Autodesk Fusion 360 part; units mm, degrees
(part 3 of 8)
  spline S114 degree 5 poles (48.8425, -65.8666) (48.8377, -65.8463) (48.8283, -65.8055) (48.814, -65.7444) (48.7948, -65.663) (48.7704, -65.5615) (48.7458, -65.4601) (48.7208, -65.3589) (48.6955, -65.2578) (48.6699, -65.1568) (48.644, -65.0561) (48.6178, -64.9555) (48.5912, -64.855) (48.5643, -64.7547) (48.5371, -64.6546) (48.5096, -64.5547) (48.4817, -64.4549) (48.4535, -64.3553) (48.4249, -64.2559) (48.396, -64.1566) (48.3668, -64.0575) (48.3373, -63.9587) (48.3074, -63.86) (48.2771, -63.7614) (48.2465, -63.6631) (48.2156, -63.565) (48.1842, -63.467) (48.1526, -63.3693) (48.1206, -63.2717) (48.0882, -63.1744) (48.0554, -63.0772) (48.0223, -62.9803) (47.9888, -62.8835) (47.9549, -62.787) (47.9207, -62.6907) (47.8861, -62.5946) (47.851, -62.4988) (47.8156, -62.4032) (47.7852, -62.322) (47.7617, -62.2601) (47.7453, -62.2173) (47.7362, -62.1935) (47.7343, -62.1887) knots -1 -1 -1 -1 -1 -1 -0.985714 -0.971429 -0.957143 -0.942857 -0.928571 -0.914286 -0.9 -0.885714 -0.871429 -0.857143 -0.842857 -0.828571 -0.814286 -0.8 -0.785714 -0.771429 -0.757143 -0.742857 -0.728571 -0.714286 -0.7 -0.685714 -0.671429 -0.657143 -0.642857 -0.628571 -0.614286 -0.6 -0.585714 -0.571429 -0.557143 -0.542857 -0.528571 -0.514286 -0.5 -0.485714 -0.471429 -0.467834 -0.467834 -0.467834 -0.467834 -0.467834 -0.467834
  spline S115 degree 3 poles (48.0492, -61.0441) (47.9469, -61.1247) (47.8613, -61.2244) (47.7331, -61.4511) (47.6918, -61.5759) (47.6653, -61.7866) (47.6651, -61.869) (47.6849, -62.0321) (47.7049, -62.1121) (47.7343, -62.1887) knots 0 0 0 0 0.039064 0.039064 0.078129 0.078129 0.102767 0.102767 0.127404 0.127404 0.127404 0.127404
  arc A58 (48.0492, -61.0441) -> (48.1406, -60.9721) centre (0, 0) ccw
  spline S116 degree 3 poles (49.3271, -60.9331) (49.2198, -60.8593) (49.0992, -60.8071) (48.8446, -60.752) (48.7132, -60.7496) (48.5041, -60.7868) (48.4254, -60.8111) (48.2756, -60.8784) (48.2051, -60.9212) (48.1406, -60.9721) knots 0 0 0 0 0.039064 0.039064 0.078129 0.078129 0.102767 0.102767 0.127404 0.127404 0.127404 0.127404
  spline S117 degree 5 poles (49.3271, -60.9331) (49.3313, -60.936) (49.3523, -60.9504) (49.3901, -60.9764) (49.4448, -61.0137) (49.5166, -61.0622) (49.6013, -61.119) (49.6864, -61.1754) (49.7717, -61.2315) (49.8574, -61.2873) (49.9433, -61.3427) (50.0295, -61.3979) (50.1161, -61.4527) (50.2029, -61.5073) (50.29, -61.5615) (50.3774, -61.6154) (50.465, -61.669) (50.553, -61.7223) (50.6412, -61.7753) (50.7296, -61.828) (50.8184, -61.8804) (50.9074, -61.9325) (50.9966, -61.9844) (51.0861, -62.0359) (51.1759, -62.0872) (51.2659, -62.1381) (51.3562, -62.1888) (51.4467, -62.2392) (51.5374, -62.2893) (51.6284, -62.3392) (51.7197, -62.3887) (51.8111, -62.438) (51.9028, -62.487) (51.9948, -62.5357) (52.0869, -62.5842) (52.1793, -62.6324) (52.2719, -62.6803) (52.3648, -62.7279) (52.4579, -62.7753) (52.5325, -62.813) (52.5886, -62.8411) (52.626, -62.8599) (52.6447, -62.8692) knots 0.467834 0.467834 0.467834 0.467834 0.467834 0.467834 0.471429 0.485714 0.5 0.514286 0.528571 0.542857 0.557143 0.571429 0.585714 0.6 0.614286 0.628571 0.642857 0.657143 0.671429 0.685714 0.7 0.714286 0.728571 0.742857 0.757143 0.771429 0.785714 0.8 0.814286 0.828571 0.842857 0.857143 0.871429 0.885714 0.9 0.914286 0.928571 0.942857 0.957143 0.971429 0.985714 1 1 1 1 1 1
  arc A59 (52.6447, -62.8692) -> (53.8597, -61.8315) centre (0, 0) ccw
  spline S118 degree 5 poles (53.8597, -61.8315) (53.8534, -61.8115) (53.8408, -61.7716) (53.8218, -61.7118) (53.7962, -61.6322) (53.764, -61.5329) (53.7315, -61.4338) (53.6986, -61.3348) (53.6655, -61.236) (53.632, -61.1374) (53.5983, -61.039) (53.5642, -60.9407) (53.5299, -60.8427) (53.4952, -60.7448) (53.4602, -60.6471) (53.4249, -60.5497) (53.3893, -60.4524) (53.3534, -60.3553) (53.3171, -60.2584) (53.2805, -60.1617) (53.2436, -60.0653) (53.2064, -59.969) (53.1688, -59.8729) (53.1309, -59.7771) (53.0927, -59.6815) (53.0542, -59.5861) (53.0153, -59.4909) (52.976, -59.3959) (52.9365, -59.3012) (52.8965, -59.2067) (52.8563, -59.1124) (52.8156, -59.0183) (52.7747, -58.9245) (52.7333, -58.831) (52.6916, -58.7377) (52.6496, -58.6446) (52.6071, -58.5518) (52.5643, -58.4592) (52.5276, -58.3807) (52.4993, -58.3209) (52.4796, -58.2795) (52.4687, -58.2565) (52.4665, -58.2518) knots -1 -1 -1 -1 -1 -1 -0.985714 -0.971429 -0.957143 -0.942857 -0.928571 -0.914286 -0.9 -0.885714 -0.871429 -0.857143 -0.842857 -0.828571 -0.814286 -0.8 -0.785714 -0.771429 -0.757143 -0.742857 -0.728571 -0.714286 -0.7 -0.685714 -0.671429 -0.657143 -0.642857 -0.628571 -0.614286 -0.6 -0.585714 -0.571429 -0.557143 -0.542857 -0.528571 -0.514286 -0.5 -0.485714 -0.471429 -0.467834 -0.467834 -0.467834 -0.467834 -0.467834 -0.467834
  spline S119 degree 3 poles (52.6906, -57.0861) (52.5949, -57.1744) (52.5174, -57.2805) (52.4074, -57.5166) (52.376, -57.6443) (52.3661, -57.8564) (52.3724, -57.9386) (52.4049, -58.0996) (52.4311, -58.1777) (52.4665, -58.2518) knots 0 0 0 0 0.039064 0.039064 0.078129 0.078129 0.102767 0.102767 0.127404 0.127404 0.127404 0.127404
  arc A60 (52.6906, -57.0861) -> (52.776, -57.0071) centre (0, 0) ccw
  spline S120 degree 3 poles (53.9558, -56.8751) (53.8431, -56.8099) (53.7187, -56.7674) (53.4606, -56.7325) (53.3294, -56.7403) (53.1239, -56.7938) (53.0473, -56.8243) (52.9032, -56.9031) (52.8363, -56.9513) (52.776, -57.0071) knots 0 0 0 0 0.039064 0.039064 0.078129 0.078129 0.102767 0.102767 0.127404 0.127404 0.127404 0.127404
  spline S121 degree 5 poles (53.9558, -56.8751) (53.9602, -56.8777) (53.9823, -56.8904) (54.022, -56.9133) (54.0795, -56.9462) (54.1549, -56.9889) (54.2438, -57.0389) (54.333, -57.0885) (54.4224, -57.1377) (54.5122, -57.1866) (54.6022, -57.2351) (54.6925, -57.2834) (54.7831, -57.3312) (54.8739, -57.3788) (54.965, -57.426) (55.0564, -57.4729) (55.148, -57.5194) (55.2398, -57.5657) (55.3319, -57.6116) (55.4242, -57.6572) (55.5168, -57.7025) (55.6096, -57.7475) (55.7027, -57.7922) (55.7959, -57.8365) (55.8894, -57.8806) (55.9832, -57.9243) (56.0771, -57.9678) (56.1713, -58.0109) (56.2657, -58.0537) (56.3604, -58.0963) (56.4552, -58.1385) (56.5503, -58.1805) (56.6455, -58.2221) (56.741, -58.2635) (56.8367, -58.3046) (56.9326, -58.3454) (57.0287, -58.3859) (57.1249, -58.4261) (57.2214, -58.466) (57.2988, -58.4977) (57.3569, -58.5214) (57.3957, -58.5371) (57.4151, -58.5449) knots 0.467834 0.467834 0.467834 0.467834 0.467834 0.467834 0.471429 0.485714 0.5 0.514286 0.528571 0.542857 0.557143 0.571429 0.585714 0.6 0.614286 0.628571 0.642857 0.657143 0.671429 0.685714 0.7 0.714286 0.728571 0.742857 0.757143 0.771429 0.785714 0.8 0.814286 0.828571 0.842857 0.857143 0.871429 0.885714 0.9 0.914286 0.928571 0.942857 0.957143 0.971429 0.985714 1 1 1 1 1 1
  arc A61 (57.4151, -58.5449) -> (58.5449, -57.4151) centre (0, 0) ccw
  spline S122 degree 5 poles (58.5449, -57.4151) (58.5371, -57.3957) (58.5214, -57.3569) (58.4977, -57.2988) (58.466, -57.2214) (58.4261, -57.1249) (58.3859, -57.0287) (58.3454, -56.9326) (58.3046, -56.8367) (58.2635, -56.741) (58.2221, -56.6455) (58.1805, -56.5503) (58.1385, -56.4552) (58.0963, -56.3604) (58.0537, -56.2657) (58.0109, -56.1713) (57.9678, -56.0771) (57.9243, -55.9832) (57.8806, -55.8894) (57.8365, -55.7959) (57.7922, -55.7027) (57.7475, -55.6096) (57.7025, -55.5168) (57.6572, -55.4242) (57.6116, -55.3319) (57.5657, -55.2398) (57.5194, -55.148) (57.4729, -55.0564) (57.426, -54.965) (57.3788, -54.8739) (57.3312, -54.7831) (57.2834, -54.6925) (57.2351, -54.6022) (57.1866, -54.5122) (57.1377, -54.4224) (57.0885, -54.333) (57.0389, -54.2438) (56.9889, -54.1549) (56.9462, -54.0795) (56.9133, -54.022) (56.8904, -53.9823) (56.8777, -53.9602) (56.8751, -53.9558) knots -1 -1 -1 -1 -1 -1 -0.985714 -0.971429 -0.957143 -0.942857 -0.928571 -0.914286 -0.9 -0.885714 -0.871429 -0.857143 -0.842857 -0.828571 -0.814286 -0.8 -0.785714 -0.771429 -0.757143 -0.742857 -0.728571 -0.714286 -0.7 -0.685714 -0.671429 -0.657143 -0.642857 -0.628571 -0.614286 -0.6 -0.585714 -0.571429 -0.557143 -0.542857 -0.528571 -0.514286 -0.5 -0.485714 -0.471429 -0.467834 -0.467834 -0.467834 -0.467834 -0.467834 -0.467834
  spline S123 degree 3 poles (57.0071, -52.776) (56.9186, -52.8716) (56.8497, -52.9835) (56.7585, -53.2275) (56.7372, -53.3572) (56.744, -53.5694) (56.7567, -53.6509) (56.8018, -53.8088) (56.834, -53.8847) (56.8751, -53.9558) knots 0 0 0 0 0.039064 0.039064 0.078129 0.078129 0.102767 0.102767 0.127404 0.127404 0.127404 0.127404
  arc A62 (57.0071, -52.776) -> (57.0861, -52.6906) centre (0, 0) ccw
  spline S124 degree 3 poles (58.2518, -52.4665) (58.1343, -52.4103) (58.007, -52.3777) (57.747, -52.3631) (57.6168, -52.3812) (57.4161, -52.4507) (57.3421, -52.487) (57.2047, -52.577) (57.1418, -52.6302) (57.0861, -52.6906) knots 0 0 0 0 0.039064 0.039064 0.078129 0.078129 0.102767 0.102767 0.127404 0.127404 0.127404 0.127404
  spline S125 degree 5 poles (58.2518, -52.4665) (58.2565, -52.4687) (58.2795, -52.4796) (58.3209, -52.4993) (58.3807, -52.5276) (58.4592, -52.5643) (58.5518, -52.6071) (58.6446, -52.6496) (58.7377, -52.6916) (58.831, -52.7333) (58.9245, -52.7747) (59.0183, -52.8156) (59.1124, -52.8563) (59.2067, -52.8965) (59.3012, -52.9365) (59.3959, -52.976) (59.4909, -53.0153) (59.5861, -53.0542) (59.6815, -53.0927) (59.7771, -53.1309) (59.8729, -53.1688) (59.969, -53.2064) (60.0653, -53.2436) (60.1617, -53.2805) (60.2584, -53.3171) (60.3553, -53.3534) (60.4524, -53.3893) (60.5497, -53.4249) (60.6471, -53.4602) (60.7448, -53.4952) (60.8427, -53.5299) (60.9407, -53.5642) (61.039, -53.5983) (61.1374, -53.632) (61.236, -53.6655) (61.3348, -53.6986) (61.4338, -53.7315) (61.5329, -53.764) (61.6322, -53.7962) (61.7118, -53.8218) (61.7716, -53.8408) (61.8115, -53.8534) (61.8315, -53.8597) knots 0.467834 0.467834 0.467834 0.467834 0.467834 0.467834 0.471429 0.485714 0.5 0.514286 0.528571 0.542857 0.557143 0.571429 0.585714 0.6 0.614286 0.628571 0.642857 0.657143 0.671429 0.685714 0.7 0.714286 0.728571 0.742857 0.757143 0.771429 0.785714 0.8 0.814286 0.828571 0.842857 0.857143 0.871429 0.885714 0.9 0.914286 0.928571 0.942857 0.957143 0.971429 0.985714 1 1 1 1 1 1
  arc A63 (61.8315, -53.8597) -> (62.8692, -52.6447) centre (0, 0) ccw
  spline S126 degree 5 poles (62.8692, -52.6447) (62.8599, -52.626) (62.8411, -52.5886) (62.813, -52.5325) (62.7753, -52.4579) (62.7279, -52.3648) (62.6803, -52.2719) (62.6324, -52.1793) (62.5842, -52.0869) (62.5357, -51.9948) (62.487, -51.9028) (62.438, -51.8111) (62.3887, -51.7197) (62.3392, -51.6284) (62.2893, -51.5374) (62.2392, -51.4467) (62.1888, -51.3562) (62.1381, -51.2659) (62.0872, -51.1759) (62.0359, -51.0861) (61.9844, -50.9966) (61.9325, -50.9074) (61.8804, -50.8184) (61.828, -50.7296) (61.7753, -50.6412) (61.7223, -50.553) (61.669, -50.465) (61.6154, -50.3774) (61.5615, -50.29) (61.5073, -50.2029) (61.4527, -50.1161) (61.3979, -50.0295) (61.3427, -49.9433) (61.2873, -49.8574) (61.2315, -49.7717) (61.1754, -49.6864) (61.119, -49.6013) (61.0622, -49.5166) (61.0137, -49.4448) (60.9764, -49.3901) (60.9504, -49.3523) (60.936, -49.3313) (60.9331, -49.3271) knots -1 -1 -1 -1 -1 -1 -0.985714 -0.971429 -0.957143 -0.942857 -0.928571 -0.914286 -0.9 -0.885714 -0.871429 -0.857143 -0.842857 -0.828571 -0.814286 -0.8 -0.785714 -0.771429 -0.757143 -0.742857 -0.728571 -0.714286 -0.7 -0.685714 -0.671429 -0.657143 -0.642857 -0.628571 -0.614286 -0.6 -0.585714 -0.571429 -0.557143 -0.542857 -0.528571 -0.514286 -0.5 -0.485714 -0.471429 -0.467834 -0.467834 -0.467834 -0.467834 -0.467834 -0.467834
  spline S127 degree 3 poles (60.9721, -48.1406) (60.8914, -48.2428) (60.8314, -48.3598) (60.7597, -48.6102) (60.7487, -48.7411) (60.7721, -48.9522) (60.7912, -49.0324) (60.8485, -49.1863) (60.8865, -49.2595) (60.9331, -49.3271) knots 0 0 0 0 0.039064 0.039064 0.078129 0.078129 0.102767 0.102767 0.127404 0.127404 0.127404 0.127404
  arc A64 (60.9721, -48.1406) -> (61.0441, -48.0492) centre (0, 0) ccw
  spline S128 degree 3 poles (62.1887, -47.7343) (62.0672, -47.6876) (61.9377, -47.6651) (61.6773, -47.6709) (61.549, -47.6992) (61.3544, -47.7842) (61.2835, -47.8262) (61.1535, -47.9267) (61.0949, -47.9847) (61.0441, -48.0492) knots 0 0 0 0 0.039064 0.039064 0.078129 0.078129 0.102767 0.102767 0.127404 0.127404 0.127404 0.127404
  spline S129 degree 5 poles (62.1887, -47.7343) (62.1935, -47.7362) (62.2173, -47.7453) (62.2601, -47.7617) (62.322, -47.7852) (62.4032, -47.8156) (62.4988, -47.851) (62.5946, -47.8861) (62.6907, -47.9207) (62.787, -47.9549) (62.8835, -47.9888) (62.9803, -48.0223) (63.0772, -48.0554) (63.1744, -48.0882) (63.2717, -48.1206) (63.3693, -48.1526) (63.467, -48.1842) (63.565, -48.2156) (63.6631, -48.2465) (63.7614, -48.2771) (63.86, -48.3074) (63.9587, -48.3373) (64.0575, -48.3668) (64.1566, -48.396) (64.2559, -48.4249) (64.3553, -48.4535) (64.4549, -48.4817) (64.5547, -48.5096) (64.6546, -48.5371) (64.7547, -48.5643) (64.855, -48.5912) (64.9555, -48.6178) (65.0561, -48.644) (65.1568, -48.6699) (65.2578, -48.6955) (65.3589, -48.7208) (65.4601, -48.7458) (65.5615, -48.7704) (65.663, -48.7948) (65.7444, -48.814) (65.8055, -48.8283) (65.8463, -48.8377) (65.8666, -48.8425) knots 0.467834 0.467834 0.467834 0.467834 0.467834 0.467834 0.471429 0.485714 0.5 0.514286 0.528571 0.542857 0.557143 0.571429 0.585714 0.6 0.614286 0.628571 0.642857 0.657143 0.671429 0.685714 0.7 0.714286 0.728571 0.742857 0.757143 0.771429 0.785714 0.8 0.814286 0.828571 0.842857 0.857143 0.871429 0.885714 0.9 0.914286 0.928571 0.942857 0.957143 0.971429 0.985714 1 1 1 1 1 1
  arc A65 (65.8666, -48.8425) -> (66.8058, -47.5498) centre (0, 0) ccw
  spline S130 degree 5 poles (66.8058, -47.5498) (66.7951, -47.5318) (66.7735, -47.496) (66.741, -47.4423) (66.6976, -47.3708) (66.6431, -47.2818) (66.5883, -47.193) (66.5333, -47.1044) (66.478, -47.0161) (66.4224, -46.928) (66.3666, -46.8402) (66.3106, -46.7526) (66.2543, -46.6653) (66.1977, -46.5782) (66.1409, -46.4914) (66.0838, -46.4049) (66.0265, -46.3186) (65.9689, -46.2326) (65.911, -46.1468) (65.8529, -46.0614) (65.7945, -45.9762) (65.7358, -45.8913) (65.6768, -45.8066) (65.6176, -45.7223) (65.5581, -45.6382) (65.4984, -45.5544) (65.4383, -45.471) (65.378, -45.3878) (65.3174, -45.3049) (65.2565, -45.2223) (65.1954, -45.1401) (65.1339, -45.0581) (65.0721, -44.9764) (65.0101, -44.8951) (64.9478, -44.8141) (64.8852, -44.7334) (64.8222, -44.6531) (64.759, -44.5731) (64.705, -44.5053) (64.6635, -44.4537) (64.6347, -44.4181) (64.6186, -44.3983) (64.6154, -44.3943) knots -1 -1 -1 -1 -1 -1 -0.985714 -0.971429 -0.957143 -0.942857 -0.928571 -0.914286 -0.9 -0.885714 -0.871429 -0.857143 -0.842857 -0.828571 -0.814286 -0.8 -0.785714 -0.771429 -0.757143 -0.742857 -0.728571 -0.714286 -0.7 -0.685714 -0.671429 -0.657143 -0.642857 -0.628571 -0.614286 -0.6 -0.585714 -0.571429 -0.557143 -0.542857 -0.528571 -0.514286 -0.5 -0.485714 -0.471429 -0.467834 -0.467834 -0.467834 -0.467834 -0.467834 -0.467834
  spline S131 degree 3 poles (64.5612, -43.2084) (64.4888, -43.3166) (64.4382, -43.4379) (64.3863, -43.6932) (64.3856, -43.8246) (64.4255, -44.0332) (64.4508, -44.1116) (64.52, -44.2606) (64.5637, -44.3305) (64.6154, -44.3943) knots 0 0 0 0 0.039064 0.039064 0.078129 0.078129 0.102767 0.102767 0.127404 0.127404 0.127404 0.127404
  arc A66 (64.5612, -43.2084) -> (64.6259, -43.1116) centre (0, 0) ccw
  spline S132 degree 3 poles (65.7422, -42.7079) (65.6174, -42.6709) (65.4865, -42.6586) (65.2274, -42.6848) (65.1017, -42.7231) (64.9143, -42.8231) (64.8469, -42.8706) (64.7253, -42.9809) (64.6714, -43.0433) (64.6259, -43.1116) knots 0 0 0 0 0.039064 0.039064 0.078129 0.078129 0.102767 0.102767 0.127404 0.127404 0.127404 0.127404
  spline S133 degree 5 poles (65.7422, -42.7079) (65.7471, -42.7094) (65.7716, -42.7166) (65.8155, -42.7296) (65.8791, -42.7481) (65.9624, -42.7721) (66.0605, -42.7999) (66.1588, -42.8273) (66.2573, -42.8543) (66.356, -42.8809) (66.4549, -42.9071) (66.5539, -42.9329) (66.6532, -42.9583) (66.7526, -42.9833) (66.8522, -43.008) (66.9519, -43.0322) (67.0519, -43.0561) (67.152, -43.0797) (67.2522, -43.1028) (67.3527, -43.1256) (67.4532, -43.148) (67.554, -43.1701) (67.6549, -43.1918) (67.756, -43.2132) (67.8572, -43.2342) (67.9585, -43.2548) (68.06, -43.2752) (68.1617, -43.2951) (68.2635, -43.3147) (68.3654, -43.334) (68.4675, -43.353) (68.5697, -43.3716) (68.6721, -43.3898) (68.7746, -43.4078) (68.8772, -43.4254) (68.98, -43.4426) (69.0829, -43.4596) (69.1859, -43.4762) (69.289, -43.4925) (69.3716, -43.5053) (69.4337, -43.5147) (69.475, -43.521) (69.4957, -43.524) knots 0.467834 0.467834 0.467834 0.467834 0.467834 0.467834 0.471429 0.485714 0.5 0.514286 0.528571 0.542857 0.557143 0.571429 0.585714 0.6 0.614286 0.628571 0.642857 0.657143 0.671429 0.685714 0.7 0.714286 0.728571 0.742857 0.757143 0.771429 0.785714 0.8 0.814286 0.828571 0.842857 0.857143 0.871429 0.885714 0.9 0.914286 0.928571 0.942857 0.957143 0.971429 0.985714 1 1 1 1 1 1
  arc A67 (69.4957, -43.524) -> (70.3306, -42.1616) centre (0, 0) ccw
  spline S134 degree 5 poles (70.3306, -42.1616) (70.3185, -42.1446) (70.2941, -42.1106) (70.2576, -42.0596) (70.2087, -41.9918) (70.1473, -41.9073) (70.0857, -41.823) (70.0239, -41.7391) (69.9619, -41.6553) (69.8996, -41.5719) (69.8371, -41.4887) (69.7743, -41.4058) (69.7114, -41.3232) (69.6481, -41.2408) (69.5847, -41.1587) (69.521, -41.0769) (69.457, -40.9954) (69.3929, -40.9142) (69.3285, -40.8333) (69.2638, -40.7526) (69.1989, -40.6723) (69.1337, -40.5922) (69.0683, -40.5125) (69.0027, -40.433) (68.9368, -40.3539) (68.8706, -40.2751) (68.8042, -40.1966) (68.7376, -40.1184) (68.6706, -40.0405) (68.6035, -39.963) (68.536, -39.8857) (68.4683, -39.8088) (68.4004, -39.7323) (68.3321, -39.6561) (68.2636, -39.5802) (68.1949, -39.5047) (68.1258, -39.4296) (68.0565, -39.3548) (67.9974, -39.2915) (67.9519, -39.2433) (67.9204, -39.21) (67.9029, -39.1915) (67.8994, -39.1878) knots -1 -1 -1 -1 -1 -1 -0.985714 -0.971429 -0.957143 -0.942857 -0.928571 -0.914286 -0.9 -0.885714 -0.871429 -0.857143 -0.842857 -0.828571 -0.814286 -0.8 -0.785714 -0.771429 -0.757143 -0.742857 -0.728571 -0.714286 -0.7 -0.685714 -0.671429 -0.657143 -0.642857 -0.628571 -0.614286 -0.6 -0.585714 -0.571429 -0.557143 -0.542857 -0.528571 -0.514286 -0.5 -0.485714 -0.471429 -0.467834 -0.467834 -0.467834 -0.467834 -0.467834 -0.467834
  spline S135 degree 3 poles (67.7523, -38.0098) (67.6886, -38.1234) (67.6476, -38.2483) (67.616, -38.5068) (67.6256, -38.6379) (67.6817, -38.8427) (67.7131, -38.9189) (67.7938, -39.0619) (67.8428, -39.1282) (67.8994, -39.1878) knots 0 0 0 0 0.039064 0.039064 0.078129 0.078129 0.102767 0.102767 0.127404 0.127404 0.127404 0.127404
  arc A68 (67.7523, -38.0098) -> (67.8091, -37.9083) centre (0, 0) ccw
  spline S136 degree 3 poles (68.8904, -37.4182) (68.763, -37.391) (68.6316, -37.389) (68.3754, -37.4355) (68.253, -37.4836) (68.0741, -37.598) (68.0106, -37.6506) (67.898, -37.7701) (67.8492, -37.8366) (67.8091, -37.9083) knots 0 0 0 0 0.039064 0.039064 0.078129 0.078129 0.102767 0.102767 0.127404 0.127404 0.127404 0.127404
  spline S137 degree 5 poles (68.8904, -37.4182) (68.8954, -37.4192) (68.9203, -37.4245) (68.9652, -37.434) (69.03, -37.4475) (69.1149, -37.4649) (69.2149, -37.4849) (69.315, -37.5045) (69.4153, -37.5237) (69.5158, -37.5425) (69.6164, -37.5608) (69.7172, -37.5788) (69.8182, -37.5963) (69.9192, -37.6135) (70.0204, -37.6302) (70.1218, -37.6466) (70.2233, -37.6626) (70.3249, -37.6782) (70.4267, -37.6934) (70.5286, -37.7082) (70.6307, -37.7227) (70.7328, -37.7368) (70.8351, -37.7505) (70.9376, -37.7639) (71.0401, -37.7769) (71.1428, -37.7895) (71.2456, -37.8018) (71.3485, -37.8137) (71.4515, -37.8253) (71.5546, -37.8365) (71.6579, -37.8474) (71.7612, -37.8579) (71.8647, -37.8681) (71.9683, -37.878) (72.072, -37.8875) (72.1758, -37.8966) (72.2797, -37.9054) (72.3837, -37.9139) (72.4878, -37.9221) (72.5712, -37.9283) (72.6338, -37.9329) (72.6755, -37.9358) (72.6964, -37.9373) knots 0.467834 0.467834 0.467834 0.467834 0.467834 0.467834 0.471429 0.485714 0.5 0.514286 0.528571 0.542857 0.557143 0.571429 0.585714 0.6 0.614286 0.628571 0.642857 0.657143 0.671429 0.685714 0.7 0.714286 0.728571 0.742857 0.757143 0.771429 0.785714 0.8 0.814286 0.828571 0.842857 0.857143 0.871429 0.885714 0.9 0.914286 0.928571 0.942857 0.957143 0.971429 0.985714 1 1 1 1 1 1
  arc A69 (72.6964, -37.9373) -> (73.4218, -36.5136) centre (0, 0) ccw
  spline S138 degree 5 poles (73.4218, -36.5136) (73.4083, -36.4976) (73.3814, -36.4656) (73.3409, -36.4176) (73.2869, -36.3538) (73.2191, -36.2744) (73.1511, -36.1952) (73.0829, -36.1164) (73.0144, -36.0378) (72.9458, -35.9595) (72.877, -35.8815) (72.8079, -35.8037) (72.7386, -35.7263) (72.6692, -35.6491) (72.5995, -35.5723) (72.5295, -35.4958) (72.4594, -35.4195) (72.389, -35.3436) (72.3185, -35.2679) (72.2477, -35.1926) (72.1767, -35.1176) (72.1054, -35.0429) (72.034, -34.9686) (71.9623, -34.8945) (71.8904, -34.8208) (71.8183, -34.7474) (71.7459, -34.6743) (71.6733, -34.6016) (71.6005, -34.5292) (71.5274, -34.4572) (71.4541, -34.3855) (71.3806, -34.3142) (71.3069, -34.2432) (71.2329, -34.1726) (71.1586, -34.1023) (71.0842, -34.0324) (71.0094, -33.9629) (70.9345, -33.8938) (70.8705, -33.8353) (70.8215, -33.7908) (70.7874, -33.7601) (70.7685, -33.7431) (70.7647, -33.7396) knots -1 -1 -1 -1 -1 -1 -0.985714 -0.971429 -0.957143 -0.942857 -0.928571 -0.914286 -0.9 -0.885714 -0.871429 -0.857143 -0.842857 -0.828571 -0.814286 -0.8 -0.785714 -0.771429 -0.757143 -0.742857 -0.728571 -0.714286 -0.7 -0.685714 -0.671429 -0.657143 -0.642857 -0.628571 -0.614286 -0.6 -0.585714 -0.571429 -0.557143 -0.542857 -0.528571 -0.514286 -0.5 -0.485714 -0.471429 -0.467834 -0.467834 -0.467834 -0.467834 -0.467834 -0.467834
  spline S139 degree 3 poles (70.5256, -32.5768) (70.471, -32.695) (70.44, -32.8228) (70.4288, -33.083) (70.4486, -33.2129) (70.5206, -33.4127) (70.5579, -33.4862) (70.6496, -33.6225) (70.7036, -33.6847) (70.7647, -33.7396) knots 0 0 0 0 0.039064 0.039064 0.078129 0.078129 0.102767 0.102767 0.127404 0.127404 0.127404 0.127404
  arc A70 (70.5256, -32.5768) -> (70.5744, -32.4711) centre (0, 0) ccw
  spline S140 degree 3 poles (71.6138, -31.8977) (71.4847, -31.8807) (71.3535, -31.889) (71.1017, -31.9555) (70.9835, -32.013) (70.8142, -32.141) (70.755, -32.1984) (70.6521, -32.3264) (70.6087, -32.3965) (70.5744, -32.4711) knots 0 0 0 0 0.039064 0.039064 0.078129 0.078129 0.102767 0.102767 0.127404 0.127404 0.127404 0.127404
  spline S141 degree 5 poles (71.6138, -31.8977) (71.6189, -31.8984) (71.6442, -31.9018) (71.6896, -31.9077) (71.7553, -31.9161) (71.8413, -31.9267) (71.9425, -31.9389) (72.0439, -31.9505) (72.1454, -31.9618) (72.2471, -31.9726) (72.3488, -31.983) (72.4507, -31.993) (72.5527, -32.0026) (72.6548, -32.0117) (72.757, -32.0205) (72.8594, -32.0289) (72.9618, -32.0368) (73.0644, -32.0444) (73.167, -32.0516) (73.2698, -32.0584) (73.3726, -32.0648) (73.4756, -32.0708) (73.5786, -32.0765) (73.6818, -32.0818) (73.785, -32.0867) (73.8884, -32.0912) (73.9918, -32.0954) (74.0953, -32.0992) (74.199, -32.1027) (74.3027, -32.1058) (74.4065, -32.1085) (74.5103, -32.1109) (74.6143, -32.1129) (74.7183, -32.1146) (74.8224, -32.116) (74.9266, -32.1169) (75.0309, -32.1176) (75.1353, -32.1179) (75.2397, -32.1178) (75.3233, -32.1175) (75.386, -32.1172) (75.4279, -32.1168) (75.4488, -32.1167) knots 0.467834 0.467834 0.467834 0.467834 0.467834 0.467834 0.471429 0.485714 0.5 0.514286 0.528571 0.542857 0.557143 0.571429 0.585714 0.6 0.614286 0.628571 0.642857 0.657143 0.671429 0.685714 0.7 0.714286 0.728571 0.742857 0.757143 0.771429 0.785714 0.8 0.814286 0.828571 0.842857 0.857143 0.871429 0.885714 0.9 0.914286 0.928571 0.942857 0.957143 0.971429 0.985714 1 1 1 1 1 1
  arc A71 (75.4488, -32.1167) -> (76.0603, -30.6404) centre (0, 0) ccw
  spline S142 degree 5 poles (76.0603, -30.6404) (76.0456, -30.6255) (76.0162, -30.5957) (75.9721, -30.5511) (75.9132, -30.4917) (75.8394, -30.4179) (75.7654, -30.3443) (75.6912, -30.271) (75.6169, -30.198) (75.5423, -30.1254) (75.4675, -30.053) (75.3926, -29.9809) (75.3175, -29.9091) (75.2421, -29.8377) (75.1666, -29.7666) (75.0909, -29.6957) (75.015, -29.6252) (74.9389, -29.555) (74.8626, -29.4852) (74.7861, -29.4156) (74.7095, -29.3464) (74.6326, -29.2776) (74.5555, -29.209) (74.4783, -29.1408) (74.4008, -29.073) (74.3231, -29.0055) (74.2452, -28.9383) (74.1672, -28.8715) (74.0889, -28.8051) (74.0104, -28.739) (73.9317, -28.6733) (73.8528, -28.6079) (73.7737, -28.543) (73.6944, -28.4784) (73.6149, -28.4141) (73.5352, -28.3503) (73.4552, -28.2869) (73.3751, -28.2238) (73.3067, -28.1706) (73.2543, -28.1301) (73.218, -28.1021) (73.1978, -28.0866) (73.1937, -28.0835) knots -1 -1 -1 -1 -1 -1 -0.985714 -0.971429 -0.957143 -0.942857 -0.928571 -0.914286 -0.9 -0.885714 -0.871429 -0.857143 -0.842857 -0.828571 -0.814286 -0.8 -0.785714 -0.771429 -0.757143 -0.742857 -0.728571 -0.714286 -0.7 -0.685714 -0.671429 -0.657143 -0.642857 -0.628571 -0.614286 -0.6 -0.585714 -0.571429 -0.557143 -0.542857 -0.528571 -0.514286 -0.5 -0.485714 -0.471429 -0.467834 -0.467834 -0.467834 -0.467834 -0.467834 -0.467834
  spline S143 degree 3 poles (72.8642, -26.943) (72.819, -27.0652) (72.7981, -27.195) (72.8073, -27.4552) (72.8373, -27.5832) (72.9248, -27.7767) (72.9677, -27.8471) (73.0698, -27.9757) (73.1286, -28.0335) (73.1937, -28.0835) knots 0 0 0 0 0.039064 0.039064 0.078129 0.078129 0.102767 0.102767 0.127404 0.127404 0.127404 0.127404
  arc A72 (72.8642, -26.943) -> (72.9045, -26.8339) centre (0, 0) ccw
  spline S144 degree 3 poles (73.8957, -26.1807) (73.7657, -26.1738) (73.6356, -26.1924) (73.3897, -26.2784) (73.2764, -26.345) (73.1176, -26.4859) (73.0631, -26.5478) (72.9706, -26.6835) (72.9328, -26.7568) (72.9045, -26.8339) knots 0 0 0 0 0.039064 0.039064 0.078129 0.078129 0.102767 0.102767 0.127404 0.127404 0.127404 0.127404
  spline S145 degree 5 poles (73.8957, -26.1807) (73.9008, -26.1809) (73.9263, -26.1823) (73.9721, -26.1846) (74.0382, -26.1878) (74.1248, -26.1917) (74.2267, -26.1959) (74.3286, -26.1995) (74.4307, -26.2028) (74.5329, -26.2056) (74.6352, -26.208) (74.7375, -26.2099) (74.8399, -26.2115) (74.9424, -26.2126) (75.045, -26.2133) (75.1477, -26.2136) (75.2505, -26.2136) (75.3533, -26.2131) (75.4562, -26.2122) (75.5592, -26.2109) (75.6622, -26.2092) (75.7653, -26.2072) (75.8685, -26.2047) (75.9718, -26.2019) (76.0751, -26.1987) (76.1785, -26.1951) (76.2819, -26.1912) (76.3854, -26.1868) (76.489, -26.1821) (76.5926, -26.1771) (76.6963, -26.1717) (76.8, -26.1659) (76.9038, -26.1598) (77.0077, -26.1533) (77.1116, -26.1464) (77.2155, -26.1393) (77.3195, -26.1317) (77.4236, -26.1238) (77.5277, -26.1156) (77.611, -26.1087) (77.6735, -26.1034) (77.7152, -26.0998) (77.736, -26.098) knots 0.467834 0.467834 0.467834 0.467834 0.467834 0.467834 0.471429 0.485714 0.5 0.514286 0.528571 0.542857 0.557143 0.571429 0.585714 0.6 0.614286 0.628571 0.642857 0.657143 0.671429 0.685714 0.7 0.714286 0.728571 0.742857 0.757143 0.771429 0.785714 0.8 0.814286 0.828571 0.842857 0.857143 0.871429 0.885714 0.9 0.914286 0.928571 0.942857 0.957143 0.971429 0.985714 1 1 1 1 1 1
  arc A73 (77.736, -26.098) -> (78.2298, -24.5784) centre (0, 0) ccw
  spline S146 degree 5 poles (78.2298, -24.5784) (78.214, -24.5646) (78.1824, -24.5372) (78.135, -24.4962) (78.0716, -24.4417) (77.9922, -24.3738) (77.9127, -24.3063) (77.8329, -24.239) (77.7531, -24.1721) (77.673, -24.1055) (77.5928, -24.0392) (77.5125, -23.9733) (77.4319, -23.9076) (77.3512, -23.8423) (77.2704, -23.7773) (77.1893, -23.7126) (77.1081, -23.6483) (77.0268, -23.5843) (76.9452, -23.5206) (76.8635, -23.4573) (76.7817, -23.3943) (76.6996, -23.3317) (76.6174, -23.2694) (76.535, -23.2075) (76.4525, -23.1459) (76.3697, -23.0847) (76.2868, -23.0239) (76.2038, -22.9634) (76.1205, -22.9033) (76.0371, -22.8436) (75.9535, -22.7843) (75.8697, -22.7253) (75.7858, -22.6667) (75.7016, -22.6086) (75.6173, -22.5508) (75.5328, -22.4934) (75.4482, -22.4364) (75.3633, -22.3799) (75.291, -22.3322) (75.2356, -22.2959) (75.1972, -22.2709) (75.1758, -22.257) (75.1715, -22.2542) knots -1 -1 -1 -1 -1 -1 -0.985714 -0.971429 -0.957143 -0.942857 -0.928571 -0.914286 -0.9 -0.885714 -0.871429 -0.857143 -0.842857 -0.828571 -0.814286 -0.8 -0.785714 -0.771429 -0.757143 -0.742857 -0.728571 -0.714286 -0.7 -0.685714 -0.671429 -0.657143 -0.642857 -0.628571 -0.614286 -0.6 -0.585714 -0.571429 -0.557143 -0.542857 -0.528571 -0.514286 -0.5 -0.485714 -0.471429 -0.467834 -0.467834 -0.467834 -0.467834 -0.467834 -0.467834
  spline S147 degree 3 poles (74.7535, -21.1431) (74.718, -21.2684) (74.7074, -21.3994) (74.737, -21.6582) (74.7769, -21.7834) (74.8793, -21.9695) (74.9276, -22.0363) (75.0395, -22.1565) (75.1026, -22.2095) (75.1715, -22.2542) knots 0 0 0 0 0.039064 0.039064 0.078129 0.078129 0.102767 0.102767 0.127404 0.127404 0.127404 0.127404
  arc A74 (74.7535, -21.1431) -> (74.7851, -21.0311) centre (0, 0) ccw
  spline S148 degree 3 poles (75.722, -20.3022) (75.5919, -20.3055) (75.4636, -20.3342) (75.2253, -20.4393) (75.1175, -20.5146) (74.9703, -20.6675) (74.9208, -20.7335) (74.8392, -20.876) (74.8073, -20.9521) (74.7851, -21.0311) knots 0 0 0 0 0.039064 0.039064 0.078129 0.078129 0.102767 0.102767 0.127404 0.127404 0.127404 0.127404
  spline S149 degree 5 poles (75.722, -20.3022) (75.7272, -20.302) (75.7526, -20.3014) (75.7985, -20.3001) (75.8646, -20.2981) (75.9512, -20.2952) (76.0531, -20.2913) (76.1551, -20.287) (76.2571, -20.2822) (76.3592, -20.277) (76.4613, -20.2714) (76.5635, -20.2653) (76.6658, -20.2588) (76.768, -20.2519) (76.8704, -20.2446) (76.9728, -20.2368) (77.0752, -20.2287) (77.1777, -20.2201) (77.2802, -20.2111) (77.3827, -20.2018) (77.4853, -20.192) (77.588, -20.1819) (77.6906, -20.1714) (77.7934, -20.1604) (77.8961, -20.1491) (77.9989, -20.1375) (78.1017, -20.1254) (78.2045, -20.113) (78.3074, -20.1002) (78.4103, -20.087) (78.5133, -20.0735) (78.6162, -20.0596) (78.7192, -20.0453) (78.8222, -20.0307) (78.9253, -20.0157) (79.0284, -20.0004) (79.1314, -19.9847) (79.2346, -19.9687) (79.3377, -19.9523) (79.4202, -19.939) (79.4821, -19.9288) (79.5234, -19.9219) (79.544, -19.9185) knots 0.467834 0.467834 0.467834 0.467834 0.467834 0.467834 0.471429 0.485714 0.5 0.514286 0.528571 0.542857 0.557143 0.571429 0.585714 0.6 0.614286 0.628571 0.642857 0.657143 0.671429 0.685714 0.7 0.714286 0.728571 0.742857 0.757143 0.771429 0.785714 0.8 0.814286 0.828571 0.842857 0.857143 0.871429 0.885714 0.9 0.914286 0.928571 0.942857 0.957143 0.971429 0.985714 1 1 1 1 1 1
  arc A75 (79.544, -19.9185) -> (79.9171, -18.3648) centre (0, 0) ccw
  spline S150 degree 5 poles (79.9171, -18.3648) (79.9002, -18.3523) (79.8666, -18.3275) (79.816, -18.2903) (79.7486, -18.2409) (79.6641, -18.1795) (79.5795, -18.1184) (79.4948, -18.0576) (79.4099, -17.9972) (79.3249, -17.9371) (79.2397, -17.8773) (79.1544, -17.8178) (79.069, -17.7587) (78.9834, -17.6999) (78.8977, -17.6414) (78.8119, -17.5833) (78.7259, -17.5256) (78.6397, -17.4681) (78.5534, -17.4111) (78.467, -17.3544) (78.3805, -17.298) (78.2938, -17.242) (78.2069, -17.1864) (78.1199, -17.1311) (78.0328, -17.0762) (77.9455, -17.0217) (77.8581, -16.9675) (77.7706, -16.9138) (77.6828, -16.8604) (77.595, -16.8074) (77.507, -16.7548) (77.4189, -16.7026) (77.3306, -16.6508) (77.2421, -16.5994) (77.1535, -16.5484) (77.0648, -16.4978) (76.9759, -16.4477) (76.8869, -16.398) (76.8111, -16.3561) (76.753, -16.3242) (76.7127, -16.3023) (76.6903, -16.2902) (76.6858, -16.2877) knots -1 -1 -1 -1 -1 -1 -0.985714 -0.971429 -0.957143 -0.942857 -0.928571 -0.914286 -0.9 -0.885714 -0.871429 -0.857143 -0.842857 -0.828571 -0.814286 -0.8 -0.785714 -0.771429 -0.757143 -0.742857 -0.728571 -0.714286 -0.7 -0.685714 -0.671429 -0.657143 -0.642857 -0.628571 -0.614286 -0.6 -0.585714 -0.571429 -0.557143 -0.542857 -0.528571 -0.514286 -0.5 -0.485714 -0.471429 -0.467834 -0.467834 -0.467834 -0.467834 -0.467834 -0.467834
  spline S151 degree 3 poles (76.1819, -15.2129) (76.1564, -15.3405) (76.1561, -15.472) (76.2059, -15.7276) (76.2555, -15.8494) (76.3722, -16.0268) (76.4256, -16.0896) (76.5465, -16.2007) (76.6136, -16.2486) (76.6858, -16.2877) knots 0 0 0 0 0.039064 0.039064 0.078129 0.078129 0.102767 0.102767 0.127404 0.127404 0.127404 0.127404
  arc A76 (76.1819, -15.2129) -> (76.2046, -15.0987) centre (0, 0) ccw
  spline S152 degree 3 poles (77.0815, -14.2985) (76.952, -14.312) (76.8264, -14.3508) (76.597, -14.4742) (76.4955, -14.5577) (76.3607, -14.7217) (76.3166, -14.7914) (76.2464, -14.9399) (76.2206, -15.0182) (76.2046, -15.0987) knots 0 0 0 0 0.039064 0.039064 0.078129 0.078129 0.102767 0.102767 0.127404 0.127404 0.127404 0.127404
  spline S153 degree 5 poles (77.0815, -14.2985) (77.0866, -14.298) (77.1119, -14.2953) (77.1575, -14.2905) (77.2234, -14.2833) (77.3095, -14.2736) (77.4107, -14.2617) (77.512, -14.2494) (77.6134, -14.2367) (77.7147, -14.2234) (77.8161, -14.2098) (77.9175, -14.1957) (78.0189, -14.1812) (78.1203, -14.1663) (78.2218, -14.151) (78.3232, -14.1352) (78.4247, -14.1191) (78.5262, -14.1025) (78.6277, -14.0855) (78.7292, -14.0681) (78.8307, -14.0504) (78.9322, -14.0322) (79.0338, -14.0136) (79.1353, -13.9947) (79.2369, -13.9754) (79.3384, -13.9557) (79.44, -13.9356) (79.5415, -13.9151) (79.6431, -13.8943) (79.7446, -13.8731) (79.8462, -13.8515) (79.9477, -13.8296) (80.0493, -13.8073) (80.1509, -13.7846) (80.2524, -13.7616) (80.354, -13.7383) (80.4555, -13.7146) (80.557, -13.6905) (80.6586, -13.6661) (80.7398, -13.6463) (80.8007, -13.6312) (80.8413, -13.6212) (80.8616, -13.6161) knots 0.467834 0.467834 0.467834 0.467834 0.467834 0.467834 0.471429 0.485714 0.5 0.514286 0.528571 0.542857 0.557143 0.571429 0.585714 0.6 0.614286 0.628571 0.642857 0.657143 0.671429 0.685714 0.7 0.714286 0.728571 0.742857 0.757143 0.771429 0.785714 0.8 0.814286 0.828571 0.842857 0.857143 0.871429 0.885714 0.9 0.914286 0.928571 0.942857 0.957143 0.971429 0.985714 1 1 1 1 1 1
  arc A77 (80.8616, -13.6161) -> (81.1116, -12.0379) centre (0, 0) ccw
  spline S154 degree 5 poles (81.1116, -12.0379) (81.0938, -12.0268) (81.0583, -12.0047) (81.005, -11.9716) (80.9339, -11.9277) (80.8449, -11.8731) (80.7558, -11.8188) (80.6665, -11.7649) (80.5772, -11.7113) (80.4877, -11.658) (80.3981, -11.6051) (80.3084, -11.5525) (80.2186, -11.5002) (80.1287, -11.4483) (80.0386, -11.3968) (79.9485, -11.3456) (79.8582, -11.2948) (79.7678, -11.2443) (79.6774, -11.1942) (79.5867, -11.1444) (79.496, -11.095) (79.4052, -11.046) (79.3143, -10.9973) (79.2232, -10.9491) (79.132, -10.9012) (79.0408, -10.8537) (78.9494, -10.8066) (78.8579, -10.7598) (78.7662, -10.7135) (78.6745, -10.6675) (78.5826, -10.622) (78.4907, -10.5769) (78.3986, -10.5322) (78.3064, -10.4879) (78.2141, -10.444) (78.1217, -10.4005) (78.0291, -10.3575) (77.9364, -10.3149) (77.8576, -10.2791) (77.7972, -10.252) (77.7553, -10.2333) (77.732, -10.2229) (77.7274, -10.2208) knots -1 -1 -1 -1 -1 -1 -0.985714 -0.971429 -0.957143 -0.942857 -0.928571 -0.914286 -0.9 -0.885714 -0.871429 -0.857143 -0.842857 -0.828571 -0.814286 -0.8 -0.785714 -0.771429 -0.757143 -0.742857 -0.728571 -0.714286 -0.7 -0.685714 -0.671429 -0.657143 -0.642857 -0.628571 -0.614286 -0.6 -0.585714 -0.571429 -0.557143 -0.542857 -0.528571 -0.514286 -0.5 -0.485714 -0.471429 -0.467834 -0.467834 -0.467834 -0.467834 -0.467834 -0.467834
  spline S155 degree 3 poles (77.1407, -9.1888) (77.1253, -9.3181) (77.1353, -9.4492) (77.2049, -9.7001) (77.2639, -9.8176) (77.3942, -9.9853) (77.4524, -10.0437) (77.5817, -10.145) (77.6523, -10.1875) (77.7274, -10.2208) knots 0 0 0 0 0.039064 0.039064 0.078129 0.078129 0.102767 0.102767 0.127404 0.127404 0.127404 0.127404
  arc A78 (77.1407, -9.1888) -> (77.1543, -9.0732) centre (0, 0) ccw
  spline S156 degree 3 poles (77.9657, -8.2067) (77.8377, -8.2303) (77.7155, -8.2788) (77.4965, -8.4198) (77.4019, -8.511) (77.2804, -8.6852) (77.2419, -8.758) (77.1835, -8.9116) (77.1639, -8.9917) (77.1543, -9.0732) knots 0 0 0 0 0.039064 0.039064 0.078129 0.078129 0.102767 0.102767 0.127404 0.127404 0.127404 0.127404
  spline S157 degree 5 poles (77.9657, -8.2067) (77.9708, -8.2057) (77.9958, -8.2011) (78.0409, -8.1927) (78.106, -8.1804) (78.191, -8.164) (78.2911, -8.1442) (78.3911, -8.124) (78.4911, -8.1033) (78.5911, -8.0822) (78.6911, -8.0606) (78.7911, -8.0386) (78.8911, -8.0162) (78.991, -7.9934) (79.0909, -7.9701) (79.1908, -7.9465) (79.2907, -7.9224) (79.3906, -7.8979) (79.4904, -7.873) (79.5903, -7.8477) (79.6901, -7.8221) (79.7899, -7.796) (79.8896, -7.7695) (79.9894, -7.7427) (80.0891, -7.7154) (80.1888, -7.6878) (80.2884, -7.6598) (80.3881, -7.6315) (80.4877, -7.6027) (80.5873, -7.5736) (80.6868, -7.5442) (80.7863, -7.5143) (80.8858, -7.4841) (80.9853, -7.4536) (81.0847, -7.4227) (81.1841, -7.3914) (81.2835, -7.3598) (81.3828, -7.3279) (81.4822, -7.2955) (81.5616, -7.2694) (81.6211, -7.2497) (81.6608, -7.2364) (81.6807, -7.2298) knots 0.467834 0.467834 0.467834 0.467834 0.467834 0.467834 0.471429 0.485714 0.5 0.514286 0.528571 0.542857 0.557143 0.571429 0.585714 0.6 0.614286 0.628571 0.642857 0.657143 0.671429 0.685714 0.7 0.714286 0.728571 0.742857 0.757143 0.771429 0.785714 0.8 0.814286 0.828571 0.842857 0.857143 0.871429 0.885714 0.9 0.914286 0.928571 0.942857 0.957143 0.971429 0.985714 1 1 1 1 1 1
  arc A79 (81.6807, -7.2298) -> (81.806, -5.6369) centre (0, 0) ccw
  spline S158 degree 5 poles (81.806, -5.6369) (81.7875, -5.6272) (81.7503, -5.6079) (81.6946, -5.5791) (81.6202, -5.5409) (81.5272, -5.4934) (81.4341, -5.4463) (81.3409, -5.3996) (81.2476, -5.3532) (81.1542, -5.3071) (81.0608, -5.2613) (80.9672, -5.216) (80.8736, -5.1709) (80.7799, -5.1262) (80.6861, -5.0819) (80.5922, -5.038) (80.4982, -4.9943) (80.4042, -4.9511) (80.31, -4.9082) (80.2158, -4.8658) (80.1215, -4.8236) (80.0271, -4.7819) (79.9326, -4.7405) (79.838, -4.6995) (79.7434, -4.6589) (79.6487, -4.6187) (79.5539, -4.5789) (79.459, -4.5395) (79.364, -4.5005) (79.2689, -4.4619) (79.1738, -4.4237) (79.0786, -4.386) (78.9833, -4.3486) (78.8879, -4.3117) (78.7924, -4.2752) (78.6968, -4.2391) (78.6012, -4.2035) (78.5055, -4.1683) (78.424, -4.1388) (78.3617, -4.1165) (78.3185, -4.1011) (78.2945, -4.0926) (78.2897, -4.0909) knots -1 -1 -1 -1 -1 -1 -0.985714 -0.971429 -0.957143 -0.942857 -0.928571 -0.914286 -0.9 -0.885714 -0.871429 -0.857143 -0.842857 -0.828571 -0.814286 -0.8 -0.785714 -0.771429 -0.757143 -0.742857 -0.728571 -0.714286 -0.7 -0.685714 -0.671429 -0.657143 -0.642857 -0.628571 -0.614286 -0.6 -0.585714 -0.571429 -0.557143 -0.542857 -0.528571 -0.514286 -0.5 -0.485714 -0.471429 -0.467834 -0.467834 -0.467834 -0.467834 -0.467834 -0.467834
  spline S159 degree 3 poles (77.6238, -3.1081) (77.6186, -3.2382) (77.6388, -3.3681) (77.728, -3.6128) (77.796, -3.7252) (77.939, -3.8822) (78.0016, -3.9359) (78.1385, -4.0267) (78.2122, -4.0635) (78.2897, -4.0909) knots 0 0 0 0 0.039064 0.039064 0.078129 0.078129 0.102767 0.102767 0.127404 0.127404 0.127404 0.127404
  arc A80 (77.6238, -3.1081) -> (77.6284, -2.9918) centre (0, 0) ccw
  spline S160 degree 3 poles (78.3693, -2.0643) (78.2435, -2.0979) (78.1255, -2.1558) (77.9183, -2.3135) (77.8311, -2.4119) (77.7236, -2.595) (77.6909, -2.6707) (77.6448, -2.8284) (77.6315, -2.9097) (77.6284, -2.9918) knots 0 0 0 0 0.039064 0.039064 0.078129 0.078129 0.102767 0.102767 0.127404 0.127404 0.127404 0.127404
  spline S161 degree 5 poles (78.3693, -2.0643) (78.3742, -2.0629) (78.3988, -2.0563) (78.4431, -2.0444) (78.507, -2.027) (78.5905, -2.004) (78.6887, -1.9764) (78.7868, -1.9484) (78.8849, -1.92) (78.983, -1.8911) (79.081, -1.8617) (79.1789, -1.832) (79.2768, -1.8018) (79.3746, -1.7712) (79.4724, -1.7402) (79.5702, -1.7087) (79.6679, -1.6769) (79.7655, -1.6447) (79.8631, -1.612) (79.9607, -1.579) (80.0581, -1.5455) (80.1556, -1.5117) (80.2529, -1.4775) (80.3503, -1.4429) (80.4475, -1.4079) (80.5448, -1.3726) (80.6419, -1.3369) (80.739, -1.3008) (80.8361, -1.2643) (80.9331, -1.2275) (81.03, -1.1903) (81.1269, -1.1527) (81.2237, -1.1148) (81.3205, -1.0766) (81.4172, -1.038) (81.5138, -0.999) (81.6104, -0.9597) (81.7069, -0.92) (81.8034, -0.88) (81.8805, -0.8478) (81.9383, -0.8234) (81.9768, -0.8071) (81.9961, -0.7989) knots 0.467834 0.467834 0.467834 0.467834 0.467834 0.467834 0.471429 0.485714 0.5 0.514286 0.528571 0.542857 0.557143 0.571429 0.585714 0.6 0.614286 0.628571 0.642857 0.657143 0.671429 0.685714 0.7 0.714286 0.728571 0.742857 0.757143 0.771429 0.785714 0.8 0.814286 0.828571 0.842857 0.857143 0.871429 0.885714 0.9 0.914286 0.928571 0.942857 0.957143 0.971429 0.985714 1 1 1 1 1 1
  arc A81 (81.9961, -0.7989) -> (81.9961, 0.7989) centre (0, 0) ccw
  spline S162 degree 5 poles (81.9961, 0.7989) (81.9768, 0.8071) (81.9383, 0.8234) (81.8805, 0.8478) (81.8034, 0.88) (81.7069, 0.92) (81.6104, 0.9597) (81.5138, 0.999) (81.4172, 1.038) (81.3205, 1.0766) (81.2237, 1.1148) (81.1269, 1.1527) (81.03, 1.1903) (80.9331, 1.2275) (80.8361, 1.2643) (80.739, 1.3008) (80.6419, 1.3369) (80.5448, 1.3726) (80.4475, 1.4079) (80.3503, 1.4429) (80.2529, 1.4775) (80.1556, 1.5117) (80.0581, 1.5455) (79.9607, 1.579) (79.8631, 1.612) (79.7655, 1.6447) (79.6679, 1.6769) (79.5702, 1.7087) (79.4724, 1.7402) (79.3746, 1.7712) (79.2768, 1.8018) (79.1789, 1.832) (79.081, 1.8617) (78.983, 1.8911) (78.8849, 1.92) (78.7868, 1.9484) (78.6887, 1.9764) (78.5905, 2.004) (78.507, 2.027) (78.4431, 2.0444) (78.3988, 2.0563) (78.3742, 2.0629) (78.3693, 2.0643) knots -1 -1 -1 -1 -1 -1 -0.985714 -0.971429 -0.957143 -0.942857 -0.928571 -0.914286 -0.9 -0.885714 -0.871429 -0.857143 -0.842857 -0.828571 -0.814286 -0.8 -0.785714 -0.771429 -0.757143 -0.742857 -0.728571 -0.714286 -0.7 -0.685714 -0.671429 -0.657143 -0.642857 -0.628571 -0.614286 -0.6 -0.585714 -0.571429 -0.557143 -0.542857 -0.528571 -0.514286 -0.5 -0.485714 -0.471429 -0.467834 -0.467834 -0.467834 -0.467834 -0.467834 -0.467834
  spline S163 degree 3 poles (77.6284, 2.9918) (77.6334, 2.8617) (77.6638, 2.7338) (77.7718, 2.4968) (77.8485, 2.3901) (78.0034, 2.2448) (78.07, 2.1962) (78.2135, 2.1164) (78.2899, 2.0855) (78.3693, 2.0643) knots 0 0 0 0 0.039064 0.039064 0.078129 0.078129 0.102767 0.102767 0.127404 0.127404 0.127404 0.127404
  arc A82 (77.6284, 2.9918) -> (77.6238, 3.1081) centre (0, 0) ccw
  spline S164 degree 3 poles (78.2897, 4.0909) (78.1669, 4.0475) (78.0538, 3.9805) (77.8596, 3.807) (77.7804, 3.7021) (77.6876, 3.5111) (77.661, 3.4331) (77.6274, 3.2723) (77.6205, 3.1901) (77.6238, 3.1081) knots 0 0 0 0 0.039064 0.039064 0.078129 0.078129 0.102767 0.102767 0.127404 0.127404 0.127404 0.127404
  spline S165 degree 5 poles (78.2897, 4.0909) (78.2945, 4.0926) (78.3185, 4.1011) (78.3617, 4.1165) (78.424, 4.1388) (78.5055, 4.1683) (78.6012, 4.2035) (78.6968, 4.2391) (78.7924, 4.2752) (78.8879, 4.3117) (78.9833, 4.3486) (79.0786, 4.386) (79.1738, 4.4237) (79.2689, 4.4619) (79.364, 4.5005) (79.459, 4.5395) (79.5539, 4.5789) (79.6487, 4.6187) (79.7434, 4.6589) (79.838, 4.6995) (79.9326, 4.7405) (80.0271, 4.7819) (80.1215, 4.8236) (80.2158, 4.8658) (80.31, 4.9082) (80.4042, 4.9511) (80.4982, 4.9943) (80.5922, 5.038) (80.6861, 5.0819) (80.7799, 5.1262) (80.8736, 5.1709) (80.9672, 5.216) (81.0608, 5.2613) (81.1542, 5.3071) (81.2476, 5.3532) (81.3409, 5.3996) (81.4341, 5.4463) (81.5272, 5.4934) (81.6202, 5.5409) (81.6946, 5.5791) (81.7503, 5.6079) (81.7875, 5.6272) (81.806, 5.6369) knots 0.467834 0.467834 0.467834 0.467834 0.467834 0.467834 0.471429 0.485714 0.5 0.514286 0.528571 0.542857 0.557143 0.571429 0.585714 0.6 0.614286 0.628571 0.642857 0.657143 0.671429 0.685714 0.7 0.714286 0.728571 0.742857 0.757143 0.771429 0.785714 0.8 0.814286 0.828571 0.842857 0.857143 0.871429 0.885714 0.9 0.914286 0.928571 0.942857 0.957143 0.971429 0.985714 1 1 1 1 1 1
  arc A83 (81.806, 5.6369) -> (81.6807, 7.2298) centre (0, 0) ccw
  spline S166 degree 5 poles (81.6807, 7.2298) (81.6608, 7.2364) (81.6211, 7.2497) (81.5616, 7.2694) (81.4822, 7.2955) (81.3828, 7.3279) (81.2835, 7.3598) (81.1841, 7.3914) (81.0847, 7.4227) (80.9853, 7.4536) (80.8858, 7.4841) (80.7863, 7.5143) (80.6868, 7.5442) (80.5873, 7.5736) (80.4877, 7.6027) (80.3881, 7.6315) (80.2884, 7.6598) (80.1888, 7.6878) (80.0891, 7.7154) (79.9894, 7.7427) (79.8896, 7.7695) (79.7899, 7.796) (79.6901, 7.8221) (79.5903, 7.8477) (79.4904, 7.873) (79.3906, 7.8979) (79.2907, 7.9224) (79.1908, 7.9465) (79.0909, 7.9701) (78.991, 7.9934) (78.8911, 8.0162) (78.7911, 8.0386) (78.6911, 8.0606) (78.5911, 8.0822) (78.4911, 8.1033) (78.3911, 8.124) (78.2911, 8.1442) (78.191, 8.164) (78.106, 8.1804) (78.0409, 8.1927) (77.9958, 8.2011) (77.9708, 8.2057) (77.9657, 8.2067) knots -1 -1 -1 -1 -1 -1 -0.985714 -0.971429 -0.957143 -0.942857 -0.928571 -0.914286 -0.9 -0.885714 -0.871429 -0.857143 -0.842857 -0.828571 -0.814286 -0.8 -0.785714 -0.771429 -0.757143 -0.742857 -0.728571 -0.714286 -0.7 -0.685714 -0.671429 -0.657143 -0.642857 -0.628571 -0.614286 -0.6 -0.585714 -0.571429 -0.557143 -0.542857 -0.528571 -0.514286 -0.5 -0.485714 -0.471429 -0.467834 -0.467834 -0.467834 -0.467834 -0.467834 -0.467834
  spline S167 degree 3 poles (77.1543, 9.0732) (77.1695, 8.9439) (77.2099, 8.8188) (77.3362, 8.591) (77.421, 8.4906) (77.5868, 8.3579) (77.657, 8.3147) (77.8064, 8.2464) (77.885, 8.2216) (77.9657, 8.2067) knots 0 0 0 0 0.039064 0.039064 0.078129 0.078129 0.102767 0.102767 0.127404 0.127404 0.127404 0.127404
  arc A84 (77.1543, 9.0732) -> (77.1407, 9.1888) centre (0, 0) ccw
  spline S168 degree 3 poles (77.7274, 10.2208) (77.6084, 10.1679) (77.5009, 10.0923) (77.3209, 9.904) (77.2501, 9.7933) (77.1726, 9.5956) (77.1522, 9.5157) (77.1313, 9.3528) (77.1309, 9.2703) (77.1407, 9.1888) knots 0 0 0 0 0.039064 0.039064 0.078129 0.078129 0.102767 0.102767 0.127404 0.127404 0.127404 0.127404
  spline S169 degree 5 poles (77.7274, 10.2208) (77.732, 10.2229) (77.7553, 10.2333) (77.7972, 10.252) (77.8576, 10.2791) (77.9364, 10.3149) (78.0291, 10.3575) (78.1217, 10.4005) (78.2141, 10.444) (78.3064, 10.4879) (78.3986, 10.5322) (78.4907, 10.5769) (78.5826, 10.622) (78.6745, 10.6675) (78.7662, 10.7135) (78.8579, 10.7598) (78.9494, 10.8066) (79.0408, 10.8537) (79.132, 10.9012) (79.2232, 10.9491) (79.3143, 10.9973) (79.4052, 11.046) (79.496, 11.095) (79.5867, 11.1444) (79.6774, 11.1942) (79.7678, 11.2443) (79.8582, 11.2948) (79.9485, 11.3456) (80.0386, 11.3968) (80.1287, 11.4483) (80.2186, 11.5002) (80.3084, 11.5525) (80.3981, 11.6051) (80.4877, 11.658) (80.5772, 11.7113) (80.6665, 11.7649) (80.7558, 11.8188) (80.8449, 11.8731) (80.9339, 11.9277) (81.005, 11.9716) (81.0583, 12.0047) (81.0938, 12.0268) (81.1116, 12.0379) knots 0.467834 0.467834 0.467834 0.467834 0.467834 0.467834 0.471429 0.485714 0.5 0.514286 0.528571 0.542857 0.557143 0.571429 0.585714 0.6 0.614286 0.628571 0.642857 0.657143 0.671429 0.685714 0.7 0.714286 0.728571 0.742857 0.757143 0.771429 0.785714 0.8 0.814286 0.828571 0.842857 0.857143 0.871429 0.885714 0.9 0.914286 0.928571 0.942857 0.957143 0.971429 0.985714 1 1 1 1 1 1
  arc A85 (81.1116, 12.0379) -> (80.8616, 13.6161) centre (0, 0) ccw
  spline S170 degree 5 poles (80.8616, 13.6161) (80.8413, 13.6212) (80.8007, 13.6312) (80.7398, 13.6463) (80.6586, 13.6661) (80.557, 13.6905) (80.4555, 13.7146) (80.354, 13.7383) (80.2524, 13.7616) (80.1509, 13.7846) (80.0493, 13.8073) (79.9477, 13.8296) (79.8462, 13.8515) (79.7446, 13.8731) (79.6431, 13.8943) (79.5415, 13.9151) (79.44, 13.9356) (79.3384, 13.9557) (79.2369, 13.9754) (79.1353, 13.9947) (79.0338, 14.0136) (78.9322, 14.0322) (78.8307, 14.0504) (78.7292, 14.0681) (78.6277, 14.0855) (78.5262, 14.1025) (78.4247, 14.1191) (78.3232, 14.1352) (78.2218, 14.151) (78.1203, 14.1663) (78.0189, 14.1812) (77.9175, 14.1957) (77.8161, 14.2098) (77.7147, 14.2234) (77.6134, 14.2367) (77.512, 14.2494) (77.4107, 14.2617) (77.3095, 14.2736) (77.2234, 14.2833) (77.1575, 14.2905) (77.1119, 14.2953) (77.0866, 14.298) (77.0815, 14.2985) knots -1 -1 -1 -1 -1 -1 -0.985714 -0.971429 -0.957143 -0.942857 -0.928571 -0.914286 -0.9 -0.885714 -0.871429 -0.857143 -0.842857 -0.828571 -0.814286 -0.8 -0.785714 -0.771429 -0.757143 -0.742857 -0.728571 -0.714286 -0.7 -0.685714 -0.671429 -0.657143 -0.642857 -0.628571 -0.614286 -0.6 -0.585714 -0.571429 -0.557143 -0.542857 -0.528571 -0.514286 -0.5 -0.485714 -0.471429 -0.467834 -0.467834 -0.467834 -0.467834 -0.467834 -0.467834
  spline S171 degree 3 poles (76.2046, 15.0987) (76.2299, 14.971) (76.2799, 14.8494) (76.4238, 14.6323) (76.5162, 14.5388) (76.6919, 14.4196) (76.7652, 14.382) (76.9195, 14.3256) (76.9998, 14.307) (77.0815, 14.2985) knots 0 0 0 0 0.039064 0.039064 0.078129 0.078129 0.102767 0.102767 0.127404 0.127404 0.127404 0.127404
  arc A86 (76.2046, 15.0987) -> (76.1819, 15.2129) centre (0, 0) ccw
  spline S172 degree 3 poles (76.6858, 16.2877) (76.5714, 16.2257) (76.4701, 16.1418) (76.3055, 15.94) (76.2436, 15.824) (76.1819, 15.6209) (76.1678, 15.5397) (76.1597, 15.3756) (76.1658, 15.2934) (76.1819, 15.2129) knots 0 0 0 0 0.039064 0.039064 0.078129 0.078129 0.102767 0.102767 0.127404 0.127404 0.127404 0.127404
  spline S173 degree 5 poles (76.6858, 16.2877) (76.6903, 16.2902) (76.7127, 16.3023) (76.753, 16.3242) (76.8111, 16.3561) (76.8869, 16.398) (76.9759, 16.4477) (77.0648, 16.4978) (77.1535, 16.5484) (77.2421, 16.5994) (77.3306, 16.6508) (77.4189, 16.7026) (77.507, 16.7548) (77.595, 16.8074) (77.6828, 16.8604) (77.7706, 16.9138) (77.8581, 16.9675) (77.9455, 17.0217) (78.0328, 17.0762) (78.1199, 17.1311) (78.2069, 17.1864) (78.2938, 17.242) (78.3805, 17.298) (78.467, 17.3544) (78.5534, 17.4111) (78.6397, 17.4681) (78.7259, 17.5256) (78.8119, 17.5833) (78.8977, 17.6414) (78.9834, 17.6999) (79.069, 17.7587) (79.1544, 17.8178) (79.2397, 17.8773) (79.3249, 17.9371) (79.4099, 17.9972) (79.4948, 18.0576) (79.5795, 18.1184) (79.6641, 18.1795) (79.7486, 18.2409) (79.816, 18.2903) (79.8666, 18.3275) (79.9002, 18.3523) (79.9171, 18.3648) knots 0.467834 0.467834 0.467834 0.467834 0.467834 0.467834 0.471429 0.485714 0.5 0.514286 0.528571 0.542857 0.557143 0.571429 0.585714 0.6 0.614286 0.628571 0.642857 0.657143 0.671429 0.685714 0.7 0.714286 0.728571 0.742857 0.757143 0.771429 0.785714 0.8 0.814286 0.828571 0.842857 0.857143 0.871429 0.885714 0.9 0.914286 0.928571 0.942857 0.957143 0.971429 0.985714 1 1 1 1 1 1
  arc A87 (79.9171, 18.3648) -> (79.544, 19.9185) centre (0, 0) ccw